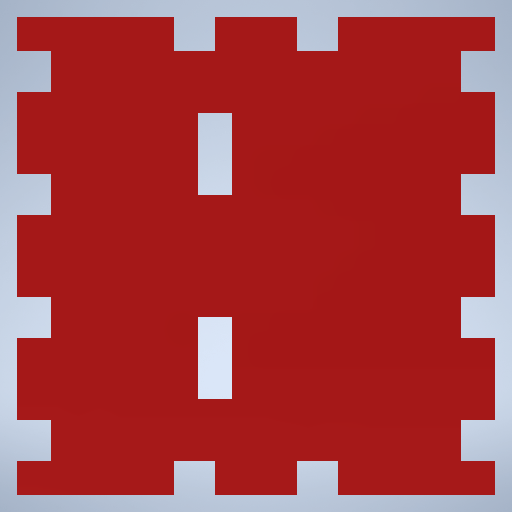
# Autodesk Inventor part: 1
Saved by Autodesk Inventor 2025.3 (Build 293356000, 356)
## iProperties
Created: 2025-12-22
Part Number: 1
Material: Generic
Document SubType Name: Sheet Metal
Designer: Balint
Density: 1 g/cm^3
Sheet Metal Rule: Default_mm
Appearance: Plywood - Weathered
Flat Pattern Width: 25 cm
Flat Pattern Length: 25 cm
Flat Pattern Area: 625 cm^2
Sheet Metal Width: 250.000 mm
Sheet Metal Length: 250.000 mm
Sheet Metal Area: 62500.000 mm^2
Author: Balint
Autodesk Inventor part; units mm, degrees
ref_plane "YZ Plane" through (0, 0, 0) normal (1, 0, 0) x (0, 1, 0)
ref_plane "XZ Plane" through (0, 0, 0) normal (0, 1, 0) x (-1, 0, 0)
ref_plane "XY Plane" through (0, 0, 0) normal (0, 0, 1) x (1, 0, 0)
sketch "Sketch1" plane through (0, 0, 0) normal (0, 0, 1) x (1, 0, 0)
  line L0 (-232, 103.6) -> (18, 103.6)
  line L1 (18, 103.6) -> (18, -146.4)
  line L2 (18, -146.4) -> (-232, -146.4)
  line L3 (-232, -146.4) -> (-232, 103.6)
  line L4 (0, -128.4) -> (0, 85.6)
  line L5 (0, -128.4) -> (-214, -128.4)
  line L6 (-214, -128.4) -> (0, -128.4)
  line L7 (18, 85.6) -> (18, 64.2)
  line L8 (18, 64.2) -> (0, 64.2)
  line L9 (0, 64.2) -> (0, 85.6)
  line L10 (18, 21.4) -> (0, 21.4)
  line L11 (0, 21.4) -> (0, 0)
  line L12 (0, 0) -> (18, 0)
  line L13 (0, -42.8) -> (18, -42.8)
  line L14 (18, -64.2) -> (0, -64.2)
  line L15 (18, -107) -> (0, -107)
  line L16 (-232, 103.6) -> (-232, 85.6)
  line L17 (0, 85.6) -> (0, 103.6)
  line L18 (-232, -107) -> (-214, -107)
  line L19 (-232, -64.2) -> (-214, -64.2)
  line L20 (-214, -42.8) -> (-232, -42.8)
  line L21 (-214, 0) -> (-232, 0)
  line L22 (-232, 21.4) -> (-214, 21.4)
  line L23 (-232, 64.2) -> (-214, 64.2)
  line L24 (-85.6, -128.4) -> (-85.6, -146.4)
  line L25 (-128.4, -128.4) -> (-128.4, -146.4)
  line L26 (-149.8, -146.4) -> (-149.8, -128.4)
  line L27 (-192.6, -146.4) -> (-192.6, -128.4)
  line L28 (-64.2, -146.4) -> (-64.2, -128.4)
  line L29 (-21.4, -146.4) -> (-21.4, -128.4)
  line L30 (-85.6, 103.6) -> (-85.6, 85.6)
  line L31 (-64.2, 85.6) -> (-64.2, 103.6)
  line L32 (-21.4, 85.6) -> (-21.4, 103.6)
  line L33 (-149.8, 85.6) -> (-149.8, 103.6)
  line L34 (-192.6, 85.6) -> (-192.6, 103.6)
  line L35 (-128.4, 103.6) -> (-128.4, 85.6)
  line L36 (0, 85.6) -> (-214, 85.6)
  line L37 (-214, 85.6) -> (-214, -128.4)
  line L38 (0, 85.6) -> (18, 85.6)
  line L39 (18, 85.6) -> (18, 103.6)
  line L40 (18, 103.6) -> (0, 103.6)
  line L41 (0, 103.6) -> (0, 85.6)
  line L42 (0, -128.4) -> (18, -128.4)
  line L43 (18, -128.4) -> (18, -146.4)
  line L44 (18, -146.4) -> (0, -146.4)
  line L45 (0, -146.4) -> (0, -128.4)
  line L46 (-214, -128.4) -> (-232, -128.4)
  line L47 (-232, -128.4) -> (-232, -146.4)
  line L48 (-232, -146.4) -> (-214, -146.4)
  line L49 (-214, -146.4) -> (-214, -128.4)
  line L50 (-214, 85.6) -> (-232, 85.6)
  line L51 (-232, 85.6) -> (-232, 103.6)
  line L52 (-232, 103.6) -> (-214, 103.6)
  line L53 (-214, 103.6) -> (-214, 85.6)
  point P0 (0, 0)
  point P1 (248.5081, 104.1116)
  point P2 (266.5081, 104.1116)
  point P3 (248.5081, 146.9116)
  point P4 (227.1081, 168.3116)
  point P5 (227.1081, 186.3116)
  point P6 (184.3081, 186.3116)
  point P7 (184.3081, 168.3116)
  point P8 (162.9081, 168.3116)
  point P9 (162.9081, 186.3116)
  point P10 (120.1081, 186.3116)
  point P11 (120.1081, 168.3116)
  point P12 (98.7081, 168.3116)
  point P13 (98.7081, 186.3116)
  point P14 (55.9081, 186.3116)
  point P15 (55.9081, 168.3116)
  point P16 (34.5081, 146.9116)
  point P17 (16.5081, 146.9116)
  point P18 (16.5081, 104.1116)
  point P19 (34.5081, 104.1116)
  point P20 (34.5081, 82.7116)
  point P21 (16.5081, 82.7116)
  point P22 (16.5081, 39.9116)
  point P23 (34.5081, 39.9116)
  point P24 (34.5081, 18.5116)
  point P25 (16.5081, 18.5116)
  point P26 (16.5081, -24.2884)
  point P27 (34.5081, -24.2884)
  point P28 (34.5081, -45.6884)
  point P29 (55.9081, -45.6884)
  point P30 (55.9081, -63.6884)
  point P31 (98.7081, -63.6884)
  point P32 (98.7081, -45.6884)
  point P33 (120.1081, -45.6884)
  point P34 (120.1081, -63.6884)
  point P35 (162.9081, -63.6884)
  point P36 (162.9081, -45.6884)
  point P37 (184.3081, -45.6884)
  point P38 (184.3081, -63.6884)
  point P39 (227.1081, -63.6884)
  point P40 (227.1081, -45.6884)
  point P41 (248.5081, -45.6884)
  point P42 (248.5081, -24.2884)
  point P43 (266.5081, -24.2884)
  point P44 (266.5081, 18.5116)
  point P45 (248.5081, 18.5116)
  point P46 (248.5081, 39.9116)
  point P47 (266.5081, 39.9116)
  point P48 (266.5081, 82.7116)
  point P49 (248.5081, 82.7116)
  dimension "d0" = 250
  dimension "d1" = 250
  dimension "d2" = 21.4
  measures "d0" distance of L1.end L2.end
  measures "d1" distance of L0.end L1.end
  measures "d2" distance of L7.start L7.end
extrude "Plate1" add sketch "Sketch1" against normal blind 18 contours L0 L53 L50 L3 | L0 L34 L36 L53 | L0 L33 L36 L34 | L36 L4 L5 L37 | L23 L37 L22 L3 | L0 L30 L36 L35 | L21 L37 L20 L3 | L0 L32 L36 L31 | L19 L37 L18 L3 | L0 L17 L36 L32 | L18 L37 L46 L3 | L0 L1 L38 L17 | L46 L49 L2 L3 | L5 L27 L2 L49 | L8 L1 L10 L4 | L5 L26 L2 L27 | L12 L1 L13 L4 | L5 L24 L2 L25 | L14 L1 L15 L4 | L5 L29 L2 L28 | L5 L45 L2 L29 | L42 L1 L2 L45
sketch "Sketch2" plane through (0, 0, 0) normal (0, 0, 1) x (1, 0, 0)
  line L0 (-232, 0) -> (-232, -42.8)
  line L1 (-128.4, 85.6) -> (-149.8, 85.6)
  line L2 (-149.8, -128.4) -> (-128.4, -128.4)
  line L3 (-128.4, 85.6) -> (-128.4, -128.4)
  line L4 (-128.4, 85.6) -> (-128.4, -21.4)
  line L5 (-137.4, 53.5) -> (-119.4, 53.5)
  line L6 (-119.4, 53.5) -> (-119.4, 10.7)
  line L7 (-119.4, 10.7) -> (-137.4, 10.7)
  line L8 (-137.4, 10.7) -> (-137.4, 53.5)
  line L9 (-137.4, 53.5) -> (-119.4, 10.7) construction
  line L10 (-119.4, 53.5) -> (-137.4, 10.7) construction
  line L11 (-128.4, -128.4) -> (-128.4, -21.4)
  line L12 (-128.4, -21.4) -> (-128.4, -74.9)
  line L13 (-137.4, -96.3) -> (-119.4, -96.3)
  line L14 (-119.4, -96.3) -> (-119.4, -53.5)
  line L15 (-119.4, -53.5) -> (-137.4, -53.5)
  line L16 (-137.4, -53.5) -> (-137.4, -96.3)
  line L17 (-137.4, -96.3) -> (-119.4, -53.5) construction
  line L18 (-119.4, -96.3) -> (-137.4, -53.5) construction
  point P0 (0, 0)
  point P1 (-232, 103.6)
  point P2 (-128.4, 32.1)
  point P3 (-232, 103.6)
  dimension "d4" = 18
  dimension "d5" = 42.8
  dimension "d6" = 42.8
  constraints: 38 end point, 7 midpoint, 4 parallel, 2 perpendicular, 1 collinear
  measures "d4" distance of L7.start L7.end
  measures "d5" distance of L5.end L7.start
  measures "d6" distance of L15.start L13.end
extrude "Cut1" cut sketch "Sketch2" against normal blind 18
sketch "Sketch3" plane through (0, 0, 0) normal (0, 0, 1) x (1, 0, 0)
  line L0 (-232, -128.4) -> (-214, -128.4) projected
  line L1 (-214, -128.4) -> (-214, -107) projected
  line L2 (-214, -128.4) -> (-214, -107) projected
  line L3 (-232, -107) -> (-214, -107) projected
  line L4 (-232, -107) -> (-232, -128.4) projected
  point P0 (0, 0)
extrude "Cut2" cut sketch "Sketch3" against normal blind 18
equation "\"d7\" = Thickness"
equation "\"d9\" = Thickness"
equation "\"d3\" = Thickness"
equation "\"BendRadius\" = Thickness"
equation "\"BendReliefWidth\" = Thickness"
equation "\"BendReliefDepth\" = 0.5 * Thickness"
equation "\"CornerReliefSize\" = 4 * Thickness"
equation "\"MinimumRemnant\" = 2 * Thickness"
equation "\"TransitionRadius\" = BendRadius"
equation "\"JacobiRadiusSize\" = BendRadius"
equation "\"GapSize\" = Thickness"
equation "\"Thickness\" = 18"
body "Solid1"
